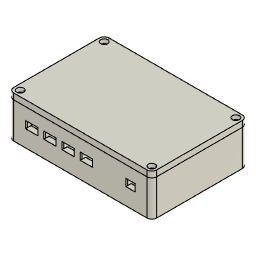
Box Innen v14 (Autodesk Fusion 360 design; units mm, degrees)
Autodesk Fusion 360 part; units mm, degrees
note: some values were not read from the file. Chosen so that the rebuilt part matches the saved one: which face or edge a step refers to.
sketch "Skizze5" plane through (0, 0, 0) normal (0, 0, 1) x (1, 0, 0)
  line L0 (60, -40) -> (-60, -40)
  line L1 (-60, -40) -> (-60, 40)
  line L2 (-60, 40) -> (60, 40)
  line L3 (60, 40) -> (60, -40)
  line L4 (60, -40) -> (-60, 40) construction
  line L5 (-60, -40) -> (60, 40) construction
  dimension "d11" = 120
  dimension "d12" = 80
  constraint perpendicular L0 L1
  constraint parallel L0 L2
  constraint parallel L1 L3
  constraint horizontal L0
  constraint coincident L4 origin
  constraint coincident L5 origin
  measures "d11" distance of L1.end L2.end
  measures "d12" distance of L0.end L1.end
extrude "Extrusion3" add sketch "Skizze5" along normal blind 30 makes body 1
sketch "Skizze6" plane through (0, 0, 30) normal (0, 0, 1) x (-1, 0, 0)
  line L0 (-60, -40) -> (60, -40)
  line L1 (60, -40) -> (60, 40)
  line L2 (60, 40) -> (-60, 40)
  line L3 (-60, 40) -> (-60, -40)
  line L4 (50.5, -38.5) -> (-50.5, -38.5)
  line L5 (-58.5, -30.5) -> (-58.5, 30.5)
  line L6 (-50.5, 38.5) -> (50.5, 38.5)
  line L7 (58.5, 30.5) -> (58.5, -30.5)
  line L8 (-50.5, -38.5) -> (-50.5, -30.5)
  line L9 (-50.5, -30.5) -> (-58.5, -30.5)
  line L10 (-58.5, 30.5) -> (-50.5, 30.5)
  line L11 (-50.5, 30.5) -> (-50.5, 38.5)
  line L12 (50.5, 38.5) -> (50.5, 30.5)
  line L13 (50.5, 30.5) -> (58.5, 30.5)
  line L14 (58.5, -30.5) -> (50.5, -30.5)
  line L15 (50.5, -30.5) -> (50.5, -38.5)
  line L16 (0, -75) -> (0, 75) construction
  line L17 (100, 0) -> (-100, 0) construction
  dimension "d15" = 1.5
  dimension "d16" = 1.5
  dimension "d26" = 8
  dimension "d27" = 8
  constraint perpendicular L1 L4
  constraint perpendicular L4 L5
  constraint perpendicular L5 L6
  constraint perpendicular L6 L7
  constraint perpendicular L4 L8
  constraint perpendicular L5 L9
  constraint perpendicular L5 L10
  constraint perpendicular L6 L12
  constraint perpendicular L7 L14
  constraint perpendicular L7 L13
  constraint perpendicular L6 L11
  constraint perpendicular L4 L15
  constraint perpendicular L6 L16
  constraint horizontal L17
  constraint symmetric L4.start L4.end L16
  constraint symmetric L5.start L7.end L16
  constraint symmetric L7.start L7.end L17
  constraint symmetric L4.start L6.end L17
  constraint symmetric L4.end L6.start L17
  constraint midpoint origin L17
  constraint midpoint origin L16
  constraint symmetric L5.start L5.end L17
  measures "d15" distance of L0 L4.end
  measures "d16" distance of L3 L5.start
  measures "d26" distance of L4.end L8.end
  measures "d27" distance of L5.start L8.end
extrude "Extrusion4" cut sketch "Skizze6" against normal blind 28 contours L4 L5 L6 L7 L8 L9 L10 L11 L12 L13 L14 L15 bodies 1
sketch "Skizze8" plane through (0, 0, 30) normal (0, 0, 1) x (-1, 0, 0)
  line L0 (58.5, 30.5) -> (58.5, -30.5)
  line L1 (58.5, -30.5) -> (50.5, -30.5)
  line L2 (50.5, -30.5) -> (50.5, -38.5)
  line L3 (50.5, -38.5) -> (-50.5, -38.5)
  line L4 (-50.5, -38.5) -> (-50.5, -30.5)
  line L5 (-50.5, -30.5) -> (-58.5, -30.5)
  line L6 (-58.5, -30.5) -> (-58.5, 30.5)
  line L7 (-58.5, 30.5) -> (-50.5, 30.5)
  line L8 (-50.5, 30.5) -> (-50.5, 38.5)
  line L9 (-50.5, 38.5) -> (50.5, 38.5)
  line L10 (50.5, 38.5) -> (50.5, 30.5)
  line L11 (50.5, 30.5) -> (58.5, 30.5)
  line L12 (-60, -40) -> (60, -40)
  line L13 (60, -40) -> (60, 40)
  line L14 (60, 40) -> (-60, 40)
  line L15 (-60, 40) -> (-60, -40)
  circle A0 centre (-55.25, -35.25) radius 1.7
  line L16 (-50.5, -30.5) -> (-60, -40) construction
  line L17 (80, 0) -> (-80, 0) construction
  line L18 (0, 55) -> (0, -55) construction
  circle A1 centre (55.25, -35.25) radius 1.7
  circle A2 centre (55.25, 35.25) radius 1.7
  circle A3 centre (-55.25, 35.25) radius 1.7
  line L19 (50.5, -30.5) -> (60, -40) construction
  line L20 (50.5, 30.5) -> (60, 40) construction
  line L21 (-50.5, 30.5) -> (-60, 40) construction
  point P0 (-55.25, -35.25)
  point P1 (55.25, -35.25)
  point P2 (55.25, 35.25)
  point P3 (-55.25, 35.25)
  dimension "d19" = 3.4
  dimension "d21" = 3.4
  dimension "d22" = 3.4
  dimension "d23" = 3.4
  constraint coincident L4.end L5.start
  constraint coincident L12.start L15.end
  constraint midpoint L16 P0
  constraint coincident P0 A0.centre
  constraint horizontal L17
  constraint perpendicular L3 L18
  constraint coincident L1.end L2.start
  constraint coincident L12.end L13.start
  constraint coincident L10.end L11.start
  constraint coincident L13.end L14.start
  constraint coincident L7.end L8.start
  constraint coincident L14.end L15.start
  constraint midpoint L19 P1
  constraint midpoint L20 P2
  constraint midpoint L21 P3
  constraint coincident P3 A3.centre
  constraint coincident P2 A2.centre
  constraint coincident P1 A1.centre
  measures "d19" diameter of A0
  measures "d21" diameter of A1
  measures "d22" diameter of A2
  measures "d23" diameter of A3
extrude "Extrusion6" cut sketch "Skizze8" against normal blind 30 contours A0 | A1 | A2 | A3 bodies 1
extrude "Extrusion7" cut sketch "Skizze8" against normal blind 28.5 contours L0 L1 L2 L3 L4 L5 L6 L7 L8 L9 L10 L11 bodies 1
sketch "Nuts" plane through (0, 0, 0) normal (0, 0, -1) x (1, 0, 0)
  line L0 (-60, -40) -> (60, -40)
  line L1 (60, -40) -> (60, 40)
  line L2 (60, 40) -> (-60, 40)
  line L3 (-60, 40) -> (-60, -40)
  line L4 (58.45, 33.4025) -> (58.45, 37.0975)
  line L5 (58.45, 37.0975) -> (55.25, 38.945)
  line L6 (55.25, 38.945) -> (52.05, 37.0975)
  line L7 (52.05, 37.0975) -> (52.05, 33.4025)
  line L8 (52.05, 33.4025) -> (55.25, 31.555)
  line L9 (55.25, 31.555) -> (58.45, 33.4025)
  line L10 (50.5, 30.5) -> (60, 40) construction
  line L11 (-55.25, 31.555) -> (-52.05, 33.4025)
  line L12 (-55.25, 38.945) -> (-58.45, 37.0975)
  line L13 (-58.45, 37.0975) -> (-58.45, 33.4025)
  line L14 (-52.05, 37.0975) -> (-55.25, 38.945)
  line L15 (-58.45, 33.4025) -> (-55.25, 31.555)
  line L16 (-52.05, 33.4025) -> (-52.05, 37.0975)
  line L17 (-58.45, -33.4025) -> (-58.45, -37.0975)
  line L18 (-55.25, -38.945) -> (-52.05, -37.0975)
  line L19 (-58.45, -37.0975) -> (-55.25, -38.945)
  line L20 (-52.05, -37.0975) -> (-52.05, -33.4025)
  line L21 (-55.25, -31.555) -> (-58.45, -33.4025)
  line L22 (-52.05, -33.4025) -> (-55.25, -31.555)
  line L23 (52.05, -37.0975) -> (55.25, -38.945)
  line L24 (58.45, -37.0975) -> (58.45, -33.4025)
  line L25 (58.45, -33.4025) -> (55.25, -31.555)
  line L26 (55.25, -31.555) -> (52.05, -33.4025)
  line L27 (52.05, -33.4025) -> (52.05, -37.0975)
  line L28 (55.25, -38.945) -> (58.45, -37.0975)
  line L29 (25, -40) -> (145, -40)
  line L30 (0, 55) -> (0, -55)
  line L31 (-100, 0) -> (100, 0)
  line L32 (0, -75) -> (0, 75)
  circle A0 centre (55.25, -35.25) radius 1.7
  circle A1 centre (55.25, 35.25) radius 1.7
  circle A2 centre (-55.25, -35.25) radius 1.7
  circle A3 centre (-55.25, 35.25) radius 1.7
  point P0 (55.25, 35.25)
  point P1 (55.25, 35.25)
  point P2 (50.5, 30.5)
  point P3 (55.25, 35.25)
  point P4 (-55.25, 35.25)
  point P5 (-55.25, 35.25)
  point P6 (-55.25, -35.25)
  point P7 (-55.25, -35.25)
  point P8 (55.25, -35.25)
  point P9 (55.25, -35.25)
  dimension "d35" = 3.2
  dimension "d36" = 3.2
  dimension "d37" = 3.2
  dimension "d38" = 3.2
  constraint coincident L1.end L2.start
  constraint midpoint L10 P3
  constraint coincident P3 P1
  constraint coincident P2 L10.start
  constraint coincident P5 P4
  constraint coincident P7 P6
  constraint coincident P9 P8
  constraint symmetric P3 P5 L30
  constraint symmetric P3 P9 L31
  constraint symmetric P5 P7 L31
  constraint parallel L27 L30
  constraint parallel L20 L32
  constraint parallel L16 L30
  constraint parallel L7 L32
  measures "d35" distance of P3 L4
  measures "d36" distance of P5 L16
  measures "d37" distance of P7 L20
  measures "d38" distance of P9 L24
extrude "Extrude8" cut sketch "Nuts" against normal blind 5 contours L4 L5 L6 L7 L8 L9 | L11 L12 L13 L14 L15 L16 | L17 L18 L19 L20 L21 L22 | L23 L24 L25 L26 L27 L28 | A0 | A1 | A2 | A3 bodies 1
sketch "Overhang long 1" plane through (0, -38.5, 0) normal (0, 1, 0) x (-1, 0, 0)
  line L0 (50.5, 30) -> (-50.5, 30)
  line L1 (-50.5, 30) -> (-50.5, 1.5)
  line L2 (-50.5, 1.5) -> (50.5, 1.5)
  line L3 (50.5, 1.5) -> (50.5, 30)
  line L4 (-50.5, 28) -> (50.5, 28)
  line L5 (50.5, 30) -> (-50.5, 30)
  dimension "d41" = 2
  constraint coincident L1 L4.start
  constraint coincident L3 L4.end
  constraint perpendicular L3 L4
  constraint coincident L0.start L3.end
  constraint coincident L0.end L1.start
  measures "d41" distance of L4.start L0.end
extrude "Extrude9" add sketch "Overhang long 1" along normal blind 3 contours L0 L1 L3 L4 L5 bodies 1
chamfer "Chamfer1" distance 2 angle 45 1 edges at (0, -35.5, 28) on bodies 1
sketch "Overhang short 1" plane through (-58.5, 0, 0) normal (1, 0, 0) x (0, 1, 0)
  line L0 (30.5, 30) -> (-30.5, 30)
  line L1 (-30.5, 30) -> (-30.5, 1.5)
  line L2 (-30.5, 1.5) -> (30.5, 1.5)
  line L3 (30.5, 1.5) -> (30.5, 30)
  line L4 (-30.5, 30) -> (30.5, 30)
  line L5 (30.5, 28) -> (-30.5, 28)
  dimension "d46" = 2
  constraint coincident L0.end L1.start
  constraint coincident L0.start L3.end
  constraint coincident L3 L5.start
  constraint coincident L1 L5.end
  constraint perpendicular L1 L5
  measures "d46" distance of L0.end L5.end
extrude "Extrude12" add sketch "Overhang short 1" along normal blind 3 contours L0 L1 L3 L4 L5 bodies 1
chamfer "Chamfer3" distance 2 angle 45 1 edges at (-55.5, 0, 28) on bodies 1
sketch "Overhang long 2" plane through (0, 38.5, 0) normal (0, -1, 0) x (1, 0, 0)
  line L0 (50.5, 30) -> (-50.5, 30)
  line L1 (-50.5, 30) -> (-50.5, 1.5)
  line L2 (-50.5, 1.5) -> (50.5, 1.5)
  line L3 (50.5, 1.5) -> (50.5, 30)
  line L4 (-50.5, 30) -> (50.5, 30)
  line L5 (50.5, 28) -> (-50.5, 28)
  dimension "d56" = 2
  constraint coincident L0.end L1.start
  constraint coincident L0.start L3.end
  constraint coincident L3 L5.start
  constraint coincident L1 L5.end
  constraint perpendicular L1 L5
  measures "d56" distance of L0.end L5.end
extrude "Extrude13" add sketch "Overhang long 2" along normal blind 3 contours L0 L1 L3 L4 L5 bodies 1
chamfer "Chamfer4" distance 2 angle 45 1 edges at (0, 35.5, 28) on bodies 1
sketch "Overhang short 2" plane through (58.5, 0, 0) normal (-1, 0, 0) x (0, -1, 0)
  line L0 (30.5, 30) -> (-30.5, 30)
  line L1 (-30.5, 30) -> (-30.5, 1.5)
  line L2 (-30.5, 1.5) -> (30.5, 1.5)
  line L3 (30.5, 1.5) -> (30.5, 30)
  line L4 (-30.5, 30) -> (30.5, 30)
  line L5 (30.5, 28) -> (-30.5, 28)
  dimension "d60" = 2
  constraint coincident L0.end L1.start
  constraint coincident L0.start L3.end
  constraint coincident L3 L5.start
  constraint coincident L1 L5.end
  constraint perpendicular L1 L5
  measures "d60" distance of L0.end L5.end
extrude "Extrude14" add sketch "Overhang short 2" along normal blind 3 contours L0 L1 L3 L4 L5 bodies 1
chamfer "Chamfer5" distance 2 angle 45 1 edges at (55.5, 0, 28) on bodies 1
sketch "Sealing" plane through (0, 0, 30) normal (0, 0, 1) x (-1, 0, 0)
  circle A0 centre (-55.25, -35.25) radius 1.7
  circle A1 centre (-55.25, 35.25) radius 1.7
  circle A2 centre (55.25, -35.25) radius 1.7
  circle A3 centre (55.25, 35.25) radius 1.7
  line L0 (55.5, -30.5) -> (50.5, -30.5)
  line L1 (50.5, -30.5) -> (50.5, -35.5)
  line L2 (50.5, -35.5) -> (-50.5, -35.5)
  line L3 (-50.5, -35.5) -> (-50.5, -30.5)
  line L4 (-50.5, -30.5) -> (-55.5, -30.5)
  line L5 (-55.5, -30.5) -> (-55.5, 30.5)
  line L6 (-55.5, 30.5) -> (-50.5, 30.5)
  line L7 (-50.5, 30.5) -> (-50.5, 35.5)
  line L8 (-50.5, 35.5) -> (50.5, 35.5)
  line L9 (50.5, 35.5) -> (50.5, 30.5)
  line L10 (50.5, 30.5) -> (55.5, 30.5)
  line L11 (55.5, 30.5) -> (55.5, -30.5)
  line L12 (-60, -40) -> (60, -40)
  line L13 (60, -40) -> (60, 40)
  line L14 (60, 40) -> (-60, 40)
  line L15 (-60, 40) -> (-60, -40)
  line L16 (50.5, -35.5) -> (-50.5, -35.5)
  line L17 (-50.5, -30.5) -> (-55.5, -30.5)
  line L18 (-55.5, 30.5) -> (-50.5, 30.5)
  line L19 (-50.5, 35.5) -> (50.5, 35.5)
  line L20 (50.5, 30.5) -> (55.5, 30.5)
  line L21 (55.5, -30.5) -> (50.5, -30.5)
  line L22 (50.5, -36.5) -> (-50.5, -36.5)
  line L23 (-50.5, -36.5) -> (-51.5, -35.5)
  line L24 (-51.5, -35.5) -> (-51.5, -31.5)
  line L25 (-51.5, -31.5) -> (-55.5, -31.5)
  line L26 (-55.5, -31.5) -> (-56.5, -30.5)
  line L27 (-56.5, -30.5) -> (-56.5, 30.5)
  line L28 (-56.5, 30.5) -> (-55.5, 31.5)
  line L29 (-55.5, 31.5) -> (-51.5, 31.5)
  line L30 (-51.5, 31.5) -> (-51.5, 35.5)
  line L31 (-51.5, 35.5) -> (-50.5, 36.5)
  line L32 (-50.5, 36.5) -> (50.5, 36.5)
  line L33 (50.5, 36.5) -> (51.5, 35.5)
  line L34 (51.5, 35.5) -> (51.5, 31.5)
  line L35 (51.5, 31.5) -> (55.5, 31.5)
  line L36 (55.5, 31.5) -> (56.5, 30.5)
  line L37 (56.5, 30.5) -> (56.5, -30.5)
  line L38 (56.5, -30.5) -> (55.5, -31.5)
  line L39 (55.5, -31.5) -> (51.5, -31.5)
  line L40 (51.5, -31.5) -> (51.5, -35.5)
  line L41 (51.5, -35.5) -> (50.5, -36.5)
  line L42 (0, -75) -> (0, 75) construction
  line L43 (100, 0) -> (-100, 0) construction
  dimension "d64" = 1
  dimension "d65" = 1
  dimension "d66" = 1
  dimension "d67" = 1
  dimension "d68" = 1
  dimension "d69" = 1
  constraint coincident L1.end L2.start
  constraint coincident L2.end L3.start
  constraint coincident L3.end L4.start
  constraint coincident L4.end L5.start
  constraint coincident L5.end L6.start
  constraint coincident L6.end L7.start
  constraint coincident L7.end L8.start
  constraint coincident L8.end L9.start
  constraint coincident L9.end L10.start
  constraint coincident L10.end L11.start
  constraint coincident L0.start L11.end
  constraint coincident L0.end L1.start
  constraint perpendicular L3 L22
  constraint perpendicular L22 L24
  constraint perpendicular L24 L25
  constraint parallel L23 L26
  constraint perpendicular L25 L27
  constraint perpendicular L27 L29
  constraint perpendicular L29 L30
  constraint parallel L28 L31
  constraint parallel L14 L32
  constraint perpendicular L14 L34
  constraint perpendicular L34 L35
  constraint parallel L33 L36
  constraint parallel L13 L37
  constraint perpendicular L36 L38
  constraint perpendicular L37 L39
  constraint perpendicular L39 L40
  constraint coincident L16 L23.end
  constraint coincident L5 L25.end
  constraint coincident L17 L26.end
  constraint vertical L42
  constraint perpendicular L37 L43
  constraint symmetric L22.start L22.end L42
  constraint symmetric L23.end L40.end L42
  constraint symmetric L25.end L38.end L42
  constraint symmetric L26.end L37.end L42
  constraint symmetric L25.end L28.end L43
  constraint symmetric L26.end L27.end L43
  constraint symmetric L23.end L30.end L43
  constraint symmetric L22.end L31.end L43
  constraint symmetric L22.start L32.end L43
  constraint symmetric L33.end L40.end L43
  constraint symmetric L35.end L38.end L43
  constraint symmetric L36.end L37.end L43
  measures "d64" distance of L2.end L22.end
  measures "d65" distance of L2.end L23.end
  measures "d66" distance of L4.end L25.end
  measures "d67" distance of L4.end L26.end
  measures "d68" distance of L1.end L40.end
  measures "d69" distance of L10.end L35.end
extrude "Extrude15" add sketch "Sealing" along normal blind 2.7 contours L22 L23 L24 L25 L26 L27 L28 L29 L30 L31 L32 L33 L34 L35 L36 L37 L38 L39 L40 L41 bodies 1
sketch "Groove" plane through (0, 0, 30) normal (0, 0, 1) x (-1, 0, 0)
  line L0 (51.5, -35.5) -> (50.5, -36.5)
  line L1 (50.5, -36.5) -> (-50.5, -36.5)
  line L2 (-50.5, -36.5) -> (-51.5, -35.5)
  line L3 (-51.5, -35.5) -> (-51.5, -31.5)
  line L4 (-51.5, -31.5) -> (-55.5, -31.5)
  line L5 (-55.5, -31.5) -> (-56.5, -30.5)
  line L6 (-56.5, -30.5) -> (-56.5, 30.5)
  line L7 (-56.5, 30.5) -> (-55.5, 31.5)
  line L8 (-55.5, 31.5) -> (-51.5, 31.5)
  line L9 (-51.5, 31.5) -> (-51.5, 35.5)
  line L10 (-51.5, 35.5) -> (-50.5, 36.5)
  line L11 (-50.5, 36.5) -> (50.5, 36.5)
  line L12 (50.5, 36.5) -> (51.5, 35.5)
  line L13 (51.5, 35.5) -> (51.5, 31.5)
  line L14 (51.5, 31.5) -> (55.5, 31.5)
  line L15 (55.5, 31.5) -> (56.5, 30.5)
  line L16 (56.5, 30.5) -> (56.5, -30.5)
  line L17 (56.5, -30.5) -> (55.5, -31.5)
  line L18 (55.5, -31.5) -> (51.5, -31.5)
  line L19 (51.5, -31.5) -> (51.5, -35.5)
  circle A0 centre (-55.25, -35.25) radius 1.7
  circle A1 centre (-55.25, 35.25) radius 1.7
  circle A2 centre (55.25, -35.25) radius 1.7
  circle A3 centre (55.25, 35.25) radius 1.7
  line L20 (-60, -40) -> (60, -40)
  line L21 (60, -40) -> (60, 40)
  line L22 (60, 40) -> (-60, 40)
  line L23 (-60, 40) -> (-60, -40)
  line L24 (50.5, -36.5) -> (-50.5, -36.5)
  line L25 (-51.5, -35.5) -> (-51.5, -31.5)
  line L26 (-55.5, -31.5) -> (-56.5, -30.5)
  line L27 (-56.5, 30.5) -> (-55.5, 31.5)
  line L28 (-51.5, 31.5) -> (-51.5, 35.5)
  line L29 (-50.5, 36.5) -> (50.5, 36.5)
  line L30 (51.5, 35.5) -> (51.5, 31.5)
  line L31 (55.5, 31.5) -> (56.5, 30.5)
  line L32 (56.5, -30.5) -> (55.5, -31.5)
  line L33 (51.5, -31.5) -> (51.5, -35.5)
  line L34 (50.9971, -37.7) -> (-50.9971, -37.7)
  line L35 (-50.9971, -37.7) -> (-52.7, -35.9971)
  line L36 (-52.7, -35.9971) -> (-52.7, -32.7)
  line L37 (-52.7, -32.7) -> (-55.9971, -32.7)
  line L38 (-55.9971, -32.7) -> (-57.7, -30.9971)
  line L39 (-57.7, -30.9971) -> (-57.7, 30.9971)
  line L40 (-57.7, 30.9971) -> (-55.9971, 32.7)
  line L41 (-55.9971, 32.7) -> (-52.7, 32.7)
  line L42 (-52.7, 32.7) -> (-52.7, 35.9971)
  line L43 (-52.7, 35.9971) -> (-50.9971, 37.7)
  line L44 (-50.9971, 37.7) -> (50.9971, 37.7)
  line L45 (50.9971, 37.7) -> (52.7, 35.9971)
  line L46 (52.7, 35.9971) -> (52.7, 32.7)
  line L47 (52.7, 32.7) -> (55.9971, 32.7)
  line L48 (55.9971, 32.7) -> (57.7, 30.9971)
  line L49 (57.7, 30.9971) -> (57.7, -30.9971)
  line L50 (57.7, -30.9971) -> (55.9971, -32.7)
  line L51 (55.9971, -32.7) -> (52.7, -32.7)
  line L52 (52.7, -32.7) -> (52.7, -35.9971)
  line L53 (52.7, -35.9971) -> (50.9971, -37.7)
  line L54 (-50.5, -30.5) -> (-52.7, -32.7) construction
  line L55 (0, -75) -> (0, 75) construction
  line L56 (100, 0) -> (-100, 0) construction
  line L57 (-100, 0) -> (-101.3533, 0) construction
  point P0 (-50.5, -30.5)
  dimension "d77" = 1.2
  dimension "d78" = 1.2
  dimension "d79" = 1.2
  dimension "d80" = 1.2
  dimension "d81" = 1.2
  dimension "d82" = 1.2
  constraint coincident L0.end L1.start
  constraint coincident L1.end L2.start
  constraint coincident L2.end L3.start
  constraint coincident L3.end L4.start
  constraint coincident L4.end L5.start
  constraint coincident L5.end L6.start
  constraint coincident L6.end L7.start
  constraint coincident L7.end L8.start
  constraint coincident L8.end L9.start
  constraint coincident L9.end L10.start
  constraint coincident L10.end L11.start
  constraint coincident L11.end L12.start
  constraint coincident L12.end L13.start
  constraint coincident L13.end L14.start
  constraint coincident L14.end L15.start
  constraint coincident L15.end L16.start
  constraint coincident L16.end L17.start
  constraint coincident L17.end L18.start
  constraint coincident L18.end L19.start
  constraint coincident L0.start L19.end
  constraint parallel L20 L34
  constraint perpendicular L36 L37
  constraint parallel L23 L39
  constraint perpendicular L23 L41
  constraint perpendicular L41 L42
  constraint parallel L40 L43
  constraint perpendicular L42 L44
  constraint perpendicular L43 L45
  constraint perpendicular L44 L46
  constraint perpendicular L46 L47
  constraint parallel L45 L48
  constraint parallel L21 L49
  constraint perpendicular L48 L50
  constraint perpendicular L21 L51
  constraint perpendicular L51 L52
  constraint collinear L3.end L36.end P0
  constraint equal L36 L37
  constraint coincident P0 L54.start
  constraint symmetric L34.end L38.end L54
  constraint vertical L55
  constraint horizontal L56
  constraint symmetric L34.start L34.end L55
  constraint symmetric L35.end L52.end L55
  constraint symmetric L37.end L50.end L55
  constraint symmetric L38.end L49.end L55
  constraint symmetric L38.end L39.end L56
  constraint symmetric L37.end L40.end L56
  constraint symmetric L35.end L42.end L56
  constraint symmetric L34.end L43.end L56
  constraint symmetric L39.end L48.end L55
  constraint symmetric L40.end L47.end L55
  constraint symmetric L42.end L45.end L55
  measures "d77" distance of L4 L37
  measures "d78" distance of L26 L38
  measures "d79" distance of L6 L39
  measures "d80" distance of L24 L34
  measures "d81" distance of L32 L50
  measures "d82" distance of L15.end L48
extrude "Extrude16" cut sketch "Groove" against normal blind 0.9 contours L34 L35 L36 L37 L38 L39 L40 L41 L42 L43 L44 L45 L46 L47 L48 L49 L50 L51 L52 L53 bodies 1
sketch "Lid Ground" plane through (0, 0, 30) normal (0, 0, 1) x (-1, 0, 0)
  line L0 (55.9971, -32.7) -> (52.7, -32.7)
  line L1 (52.7, -32.7) -> (52.7, -35.9971)
  line L2 (52.7, -35.9971) -> (50.9971, -37.7)
  line L3 (50.9971, -37.7) -> (-50.9971, -37.7)
  line L4 (-50.9971, -37.7) -> (-52.7, -35.9971)
  line L5 (-52.7, -35.9971) -> (-52.7, -32.7)
  line L6 (-52.7, -32.7) -> (-55.9971, -32.7)
  line L7 (-55.9971, -32.7) -> (-57.7, -30.9971)
  line L8 (-57.7, -30.9971) -> (-57.7, 30.9971)
  line L9 (-57.7, 30.9971) -> (-55.9971, 32.7)
  line L10 (-55.9971, 32.7) -> (-52.7, 32.7)
  line L11 (-52.7, 32.7) -> (-52.7, 35.9971)
  line L12 (-52.7, 35.9971) -> (-50.9971, 37.7)
  line L13 (-50.9971, 37.7) -> (50.9971, 37.7)
  line L14 (50.9971, 37.7) -> (52.7, 35.9971)
  line L15 (52.7, 35.9971) -> (52.7, 32.7)
  line L16 (52.7, 32.7) -> (55.9971, 32.7)
  line L17 (55.9971, 32.7) -> (57.7, 30.9971)
  line L18 (57.7, 30.9971) -> (57.7, -30.9971)
  line L19 (57.7, -30.9971) -> (55.9971, -32.7)
  circle A0 centre (-55.25, -35.25) radius 1.7
  circle A1 centre (-55.25, 35.25) radius 1.7
  circle A2 centre (55.25, -35.25) radius 1.7
  circle A3 centre (55.25, 35.25) radius 1.7
  line L20 (-60, -40) -> (60, -40)
  line L21 (60, -40) -> (60, 40)
  line L22 (60, 40) -> (-60, 40)
  line L23 (-60, 40) -> (-60, -40)
  line L24 (60, -40) -> (-60, -40)
  line L25 (-60, -40) -> (-60, 40)
  line L26 (-60, 40) -> (60, 40)
  line L27 (60, 40) -> (60, -40)
  constraint horizontal L24
  constraint vertical L25
  constraint horizontal L26
  constraint vertical L27
  constraint coincident L22.end L23.start
  constraint coincident L20.end L21.start
extrude "Extrude17" add sketch "Lid Ground" along normal blind 5 separate body makes body 2
delete_face "DeleteFace1" 20 faces at (-57.1324, 31.5647, 31.6667) (-57.7, -10.3324, 33.3333) (-56.5647, -32.1324, 31.6667) (-53.799, -32.7, 31.6667) (-52.7, -34.898, 31.6667) (-51.5647, -37.1324, 31.6667) (16.999, -37.7, 31.6667) (52.1324, -36.5647, 31.6667) (52.7, -33.799, 31.6667) (54.898, -32.7, 31.6667) (57.1324, -31.5647, 31.6667) (57.7, 10.3324, 33.3333) (56.5647, 32.1324, 31.6667) (53.799, 32.7, 31.6667) (52.7, 34.898, 31.6667) (51.5647, 37.1324, 31.6667) (-16.999, 37.7, 31.6667) (-52.1324, 36.5647, 31.6667) (-52.7, 33.799, 31.6667) (-54.898, 32.7, 31.6667) on bodies 2
sketch "Screw heads" plane through (0, 0, 35) normal (0, 0, 1) x (-1, 0, 0)
  circle A0 centre (55.25, -35.25) radius 1.7
  circle A1 centre (-55.25, 35.25) radius 1.7
  circle A2 centre (-55.25, -35.25) radius 1.7
  circle A3 centre (55.25, 35.25) radius 1.7
  line L0 (60, 40) -> (-60, 40)
  line L1 (-60, 40) -> (-60, -40)
  line L2 (-60, -40) -> (60, -40)
  line L3 (60, -40) -> (60, 40)
  circle A4 centre (55.25, -35.25) radius 2.95
  circle A5 centre (-55.25, -35.25) radius 2.95
  circle A6 centre (-55.25, 35.25) radius 2.95
  circle A7 centre (55.25, 35.25) radius 2.95
  dimension "d87" = 5.9
  dimension "d88" = 5.9
  dimension "d89" = 5.9
  dimension "d90" = 5.9
  constraint concentric A0 A4
  constraint concentric A2 A5
  constraint concentric A1 A6
  constraint concentric A3 A7
  measures "d87" diameter of A4
  measures "d88" diameter of A5
  measures "d89" diameter of A6
  measures "d90" diameter of A7
extrude "Extrude18" cut sketch "Screw heads" against normal blind 3.4 contours A4 | A5 | A6 | A7 bodies 2
sketch "Sealing groove" plane through (0, 0, 30) normal (0, 0, -1) x (1, 0, 0)
  line L0 (-60, -40) -> (60, -40)
  line L1 (60, -40) -> (60, 40)
  line L2 (60, 40) -> (-60, 40)
  line L3 (-60, 40) -> (-60, -40)
  line L4 (-50.6243, 36.8) -> (50.6243, 36.8)
  line L5 (50.6243, 36.8) -> (51.8, 35.6243)
  line L6 (51.8, 31.8) -> (55.6243, 31.8)
  line L7 (51.8, 35.6243) -> (51.8, 31.8)
  line L8 (55.6243, 31.8) -> (56.8, 30.6243)
  line L9 (56.8, 30.6243) -> (56.8, -30.6243)
  line L10 (56.8, -30.6243) -> (55.6243, -31.8)
  line L11 (55.6243, -31.8) -> (51.8, -31.8)
  line L12 (51.8, -31.8) -> (51.8, -35.6243)
  line L13 (50.6243, -36.8) -> (-50.6243, -36.8)
  line L14 (-50.6243, -36.8) -> (-51.8, -35.6243)
  line L15 (-51.8, -35.6243) -> (-51.8, -31.8)
  line L16 (-51.8, -31.8) -> (-55.6243, -31.8)
  line L17 (-56.8, -30.6243) -> (-56.8, 30.6243)
  line L18 (-56.8, 30.6243) -> (-55.6243, 31.8)
  line L19 (-51.8, 31.8) -> (-51.8, 35.6243)
  line L20 (-51.8, 35.6243) -> (-50.6243, 36.8)
  line L21 (-55.6243, 31.8) -> (-51.8, 31.8)
  line L22 (-55.6243, -31.8) -> (-56.8, -30.6243)
  line L23 (50.6243, -36.8) -> (51.8, -35.6243)
  line L24 (-100, 0) -> (100, 0) construction
  line L25 (0, -75) -> (0, 75) construction
  line L26 (-50.2, 35.2) -> (50.2, 35.2)
  line L27 (50.2, 35.2) -> (50.2, 30.2)
  line L28 (50.2, 30.2) -> (55.2, 30.2)
  line L29 (55.2, 30.2) -> (55.2, -30.2)
  line L30 (55.2, -30.2) -> (50.2, -30.2)
  line L31 (50.2, -30.2) -> (50.2, -35.2)
  line L32 (50.2, -35.2) -> (-50.2, -35.2)
  line L33 (-50.2, -35.2) -> (-50.2, -30.2)
  line L34 (-50.2, -30.2) -> (-55.2, -30.2)
  line L35 (-55.2, -30.2) -> (-55.2, 30.2)
  line L36 (-55.2, 30.2) -> (-50.2, 30.2)
  line L37 (-50.2, 30.2) -> (-50.2, 35.2)
  line L38 (-55.5, 30.5) -> (-55.5, -30.5) construction
  circle A0 centre (-55.25, -35.25) radius 1.7
  circle A1 centre (55.25, 35.25) radius 1.7
  circle A2 centre (55.25, -35.25) radius 1.7
  circle A3 centre (-55.25, 35.25) radius 1.7
  line L39 (60, 40) -> (-60, 40)
  line L40 (-60, 40) -> (-60, -40)
  line L41 (-60, -40) -> (60, -40)
  line L42 (60, -40) -> (60, 40)
  line L43 (51.5, 35.5) -> (50.5, 36.5)
  line L44 (55.5, 31.5) -> (51.5, 31.5)
  line L45 (51.5, 31.5) -> (51.5, 35.5)
  line L46 (56.5, -30.5) -> (56.5, 30.5)
  line L47 (50.5, 36.5) -> (-50.5, 36.5)
  line L48 (56.5, 30.5) -> (55.5, 31.5)
  line L49 (50.5, 35.5) -> (-50.5, 35.5)
  line L50 (55.5, 30.5) -> (50.5, 30.5)
  line L51 (50.5, 30.5) -> (50.5, 35.5) construction
  line L52 (55.5, 30.5) -> (55.5, -30.5) construction
  point P0 (55.5, 31.5)
  dimension "d101" = 0.3
  dimension "d102" = 1.6
  dimension "d104" = 0.3
  dimension "d105" = 0.3
  dimension "d106" = 0.3
  dimension "d107" = 0.3
  dimension "d108" = 0.3
  dimension "d109" = 0.3
  dimension "d110" = 0.3
  dimension "d111" = 0.3
  dimension "d112" = 0.3
  dimension "d113" = 0.3
  constraint perpendicular L6 L7
  constraint parallel L1 L9
  constraint horizontal L11
  constraint perpendicular L11 L12
  constraint perpendicular L15 L16
  constraint perpendicular L16 L17
  constraint parallel L17 L19
  constraint perpendicular L19 L21
  constraint coincident L6.start L7.end
  constraint symmetric L8.end L9.end L24
  constraint symmetric L6.end L10.end L24
  constraint symmetric L5.end L12.end L24
  constraint symmetric L4.end L13.start L24
  constraint symmetric L4.start L4.end L25
  constraint symmetric L5.end L19.end L25
  constraint symmetric L8.end L17.end L25
  constraint symmetric L6.end L25 L18.end
  constraint coincident L18.end L21.start
  constraint symmetric L9.end L17.start L25
  constraint coincident L17.start L22.end
  constraint symmetric L10.end L16.end L25
  constraint symmetric L13.start L13.end L25
  constraint symmetric L12.end L14.end L25
  constraint perpendicular L26 L27
  constraint perpendicular L27 L28
  constraint perpendicular L28 L29
  constraint perpendicular L29 L30
  constraint perpendicular L30 L31
  constraint perpendicular L31 L32
  constraint perpendicular L32 L33
  constraint perpendicular L33 L34
  constraint perpendicular L34 L35
  constraint perpendicular L33 L36
  constraint perpendicular L26 L37
  constraint symmetric L25 L27 L37
  constraint symmetric L24 L34 L36
  constraint symmetric L24 L26 L32
  constraint symmetric L24 L33 L37
  constraint symmetric L25 L28 L36
  constraint symmetric L25 L30 L34
  constraint parallel L8 L48
  constraint coincident L50.end L51.start
  constraint coincident L49.start L51.end
  constraint coincident L50.start L52.start
  constraint perpendicular L30 L52
  measures "d101" distance of L35 L38
  measures "d102" distance of L17 L35
  measures "d104" distance of L8 P0
  measures "d105" distance of L5 L43
  measures "d106" distance of L6 L44
  measures "d107" distance of L7 L45
  measures "d108" distance of L9 L46
  measures "d109" distance of L4 L47
  measures "d110" distance of L26 L49
  measures "d111" distance of L28 L50
  measures "d112" distance of L27 L51
  measures "d113" distance of L29 L52
extrude "Extrude20" cut sketch "Sealing groove" against normal blind 3 contours L4 L5 L6 L7 L8 L9 L10 L11 L12 L13 L14 L15 L16 L17 L18 L19 L20 L21 L22 L23 bodies 2
sketch "Lid inner" plane through (0, 0, 30) normal (0, 0, -1) x (1, 0, 0)
  line L0 (-50.2, 35.2) -> (-50.2, 30.2)
  line L1 (-50.2, 30.2) -> (-55.2, 30.2)
  line L2 (-55.2, 30.2) -> (-55.2, -30.2)
  line L3 (-55.2, -30.2) -> (-50.2, -30.2)
  line L4 (-50.2, -30.2) -> (-50.2, -35.2)
  line L5 (-50.2, -35.2) -> (50.2, -35.2)
  line L6 (50.2, -35.2) -> (50.2, -30.2)
  line L7 (50.2, -30.2) -> (55.2, -30.2)
  line L8 (55.2, -30.2) -> (55.2, 30.2)
  line L9 (55.2, 30.2) -> (50.2, 30.2)
  line L10 (50.2, 30.2) -> (50.2, 35.2)
  line L11 (50.2, 35.2) -> (-50.2, 35.2)
  line L12 (-49.2, 34.2) -> (49.2, 34.2)
  line L13 (49.2, 34.2) -> (49.2, 29.2)
  line L14 (49.2, 29.2) -> (54.2, 29.2)
  line L15 (54.2, 29.2) -> (54.2, -29.2)
  line L16 (54.2, -29.2) -> (49.2, -29.2)
  line L17 (49.2, -29.2) -> (49.2, -34.2)
  line L18 (49.2, -34.2) -> (-49.2, -34.2)
  line L19 (-49.2, -34.2) -> (-49.2, -29.2)
  line L20 (-49.2, -29.2) -> (-54.2, -29.2)
  line L21 (-54.2, -29.2) -> (-54.2, 29.2)
  line L22 (-54.2, 29.2) -> (-49.2, 29.2)
  line L23 (-49.2, 29.2) -> (-49.2, 34.2)
  line L24 (0, -75) -> (0, 75) construction
  line L25 (-100, 0) -> (100, 0) construction
  dimension "d118" = 1
  dimension "d119" = 1
  dimension "d120" = 1
  dimension "d121" = 1
  constraint perpendicular L0 L12
  constraint perpendicular L12 L13
  constraint perpendicular L13 L14
  constraint perpendicular L7 L15
  constraint perpendicular L15 L16
  constraint perpendicular L7 L17
  constraint perpendicular L17 L18
  constraint perpendicular L18 L19
  constraint perpendicular L19 L20
  constraint perpendicular L18 L21
  constraint perpendicular L21 L22
  constraint perpendicular L12 L23
  constraint symmetric L14 L22 L24
  constraint symmetric L20 L22 L25
  constraint symmetric L12 L18 L25
  constraint symmetric L14 L16 L25
  constraint symmetric L13 L17 L25
  constraint symmetric L19 L23 L25
  measures "d118" distance of L11 L12
  measures "d119" distance of L10 L13
  measures "d120" distance of L9 L14
  measures "d121" distance of L8 L15
extrude "Extrude21" cut sketch "Lid inner" against normal blind 3 contours L12 L13 L14 L15 L16 L17 L18 L19 L20 L21 L22 L23 bodies 2
fillet "Fillet1" radius 4 1 edges at (-60, -40, 15) on bodies 1
fillet "Fillet2" radius 4 1 edges at (-60, 40, 15) on bodies 1
fillet "Fillet3" radius 4 1 edges at (60, 40, 15) on bodies 1
fillet "Fillet4" radius 4 1 edges at (60, -40, 15) on bodies 1
fillet "Fillet5" radius 4 1 edges at (60, -40, 32.5) on bodies 2
fillet "Fillet6" radius 4 1 edges at (-60, -40, 32.5) on bodies 2
fillet "Fillet7" radius 4 1 edges at (-60, 40, 32.5) on bodies 2
fillet "Fillet8" radius 4 1 edges at (60, 40, 32.5) on bodies 2
sketch "JST XH connectors" plane through (0, -40, 0) normal (0, -1, 0) x (1, 0, 0)
  line L0 (56, 0) -> (56, 30)
  line L1 (56, 30) -> (-56, 30)
  line L2 (-56, 30) -> (-56, 0)
  line L3 (-56, 0) -> (56, 0)
  line L4 (-35.7, 13.9817) -> (-46, 13.9817)
  line L5 (-46, 13.9817) -> (-46, 19.9817)
  line L6 (-46, 19.9817) -> (-35.7, 19.9817)
  line L7 (-35.7, 19.9817) -> (-35.7, 13.9817)
  line L8 (-35.7, 13.9817) -> (-46, 19.9817) construction
  line L9 (-46, 13.9817) -> (-35.7, 19.9817) construction
  line L10 (-56, 16.9788) -> (56, 17) construction
  line L11 (-20.4, 13.9846) -> (-30.7, 13.9846)
  line L12 (-20.4, 19.9846) -> (-20.4, 13.9846)
  line L13 (-30.7, 19.9846) -> (-20.4, 19.9846)
  line L14 (-30.7, 13.9846) -> (-30.7, 19.9846)
  line L15 (-20.4, 13.9846) -> (-30.7, 19.9846) construction
  line L16 (-30.7, 13.9846) -> (-20.4, 19.9846) construction
  line L17 (-5.1, 13.9874) -> (-15.4, 13.9874)
  line L18 (-5.1, 19.9874) -> (-5.1, 13.9874)
  line L19 (-15.4, 19.9874) -> (-5.1, 19.9874)
  line L20 (-15.4, 13.9874) -> (-5.1, 19.9874) construction
  line L21 (-5.1, 13.9874) -> (-15.4, 19.9874) construction
  line L22 (-15.4, 13.9874) -> (-15.4, 19.9874)
  line L23 (10.2, 13.9903) -> (-0.1, 13.9903)
  line L24 (10.2, 19.9903) -> (10.2, 13.9903)
  line L25 (-0.1, 19.9903) -> (10.2, 19.9903)
  line L26 (-0.1, 13.9903) -> (10.2, 19.9903) construction
  line L27 (10.2, 13.9903) -> (-0.1, 19.9903) construction
  line L28 (-0.1, 13.9903) -> (-0.1, 19.9903)
  line L29 (46, 19.9974) -> (46, 13.9974)
  line L30 (38.2, 19.9974) -> (46, 19.9974)
  line L31 (38.2, 13.9974) -> (38.2, 19.9974)
  line L32 (46, 13.9974) -> (38.2, 13.9974)
  line L33 (46, 13.9974) -> (38.2, 19.9974) construction
  line L34 (38.2, 13.9974) -> (46, 19.9974) construction
  point P0 (-40.85, 16.9817)
  point P1 (-56, 16.9788)
  point P2 (56, 17)
  point P3 (-25.55, 16.9846)
  point P4 (-10.25, 16.9874)
  point P5 (5.05, 16.9903)
  point P6 (42.1, 16.9974)
  dimension "d134" = 6
  dimension "d135" = 10.3
  dimension "d136" = 10
  dimension "d138" = 6
  dimension "d139" = 10.3
  dimension "d140" = 5
  dimension "d141" = 6
  dimension "d142" = 10.3
  dimension "d143" = 6
  dimension "d144" = 10.3
  dimension "d145" = 5
  dimension "d146" = 5
  dimension "d147" = 6
  dimension "d148" = 7.8
  dimension "d149" = 10
  constraint perpendicular L4 L5
  constraint parallel L4 L6
  constraint parallel L5 L7
  constraint horizontal L4
  constraint coincident L8 P0
  constraint coincident L9 P0
  constraint midpoint L8 P0
  constraint coincident L2 P1
  constraint coincident L0 P2
  constraint coincident P1 L10.start
  constraint coincident P2 L10.end
  constraint coincident P0 L10
  constraint perpendicular L11 L14
  constraint parallel L11 L13
  constraint parallel L12 L14
  constraint horizontal L11
  constraint coincident P3 L15
  constraint coincident P3 L16
  constraint midpoint P3 L15
  constraint coincident L10 P3
  constraint perpendicular L17 L22
  constraint parallel L17 L19
  constraint parallel L18 L22
  constraint horizontal L17
  constraint coincident P4 L21
  constraint coincident P4 L20
  constraint midpoint P4 L21
  constraint perpendicular L23 L28
  constraint parallel L23 L25
  constraint parallel L24 L28
  constraint horizontal L23
  constraint coincident P5 L27
  constraint coincident P5 L26
  constraint midpoint P5 L27
  constraint coincident L10 P4
  constraint coincident L10 P5
  constraint perpendicular L31 L32
  constraint parallel L30 L32
  constraint parallel L29 L31
  constraint horizontal L32
  constraint coincident P6 L33
  constraint coincident P6 L34
  constraint midpoint P6 L33
  constraint coincident L10 P6
  measures "d134" distance of L4.end L5.end
  measures "d135" distance of L5.end L6.end
  measures "d136" distance of L2 L5
  measures "d138" distance of L13.start L11.end
  measures "d139" distance of L13.start L12.start
  measures "d140" distance of L7 L14
  measures "d141" distance of L19.start L17.end
  measures "d142" distance of L19.start L18.start
  measures "d143" distance of L25.start L23.end
  measures "d144" distance of L25.start L24.start
  measures "d145" distance of L12 L22
  measures "d146" distance of L18 L28
  measures "d147" distance of L31.start L30.start
  measures "d148" distance of L29.start L30.start
  measures "d149" distance of L0 L29
extrude "Extrude22" cut sketch "JST XH connectors" against normal blind 1.5 contours L4 L5 L6 L7 | L11 L12 L13 L14 | L17 L18 L19 L22 | L23 L24 L25 L28 | L29 L30 L31 L32 bodies 1
sketch "JST XH connector support" plane through (0, -38.5, 0) normal (0, 1, 0) x (-1, 0, 0)
  line L0 (5.1, 13.9874) -> (5.1, 19.9874)
  line L1 (5.1, 19.9874) -> (15.4, 19.9874)
  line L2 (15.4, 19.9874) -> (15.4, 13.9874)
  line L3 (15.4, 13.9874) -> (5.1, 13.9874)
  line L4 (20.4, 13.9846) -> (20.4, 19.9846)
  line L5 (20.4, 19.9846) -> (30.7, 19.9846)
  line L6 (30.7, 19.9846) -> (30.7, 13.9846)
  line L7 (30.7, 13.9846) -> (20.4, 13.9846)
  line L8 (-10.2, 13.9903) -> (-10.2, 19.9903)
  line L9 (-10.2, 19.9903) -> (0.1, 19.9903)
  line L10 (0.1, 19.9903) -> (0.1, 13.9903)
  line L11 (0.1, 13.9903) -> (-10.2, 13.9903)
  line L12 (46, 19.9817) -> (46, 13.9817)
  line L13 (46, 13.9817) -> (35.7, 13.9817)
  line L14 (35.7, 13.9817) -> (35.7, 19.9817)
  line L15 (35.7, 19.9817) -> (46, 19.9817)
  line L16 (-46, 19.9974) -> (-38.2, 19.9974)
  line L17 (-38.2, 19.9974) -> (-38.2, 13.9974)
  line L18 (-38.2, 13.9974) -> (-46, 13.9974)
  line L19 (-46, 13.9974) -> (-46, 19.9974)
  line L20 (50.5, 28) -> (-50.5, 28)
  line L21 (-50.5, 28) -> (-50.5, 1.5)
  line L22 (-50.5, 1.5) -> (50.5, 1.5)
  line L23 (50.5, 1.5) -> (50.5, 28)
  line L24 (-46, 13.9974) -> (-38.2, 13.9974)
  line L25 (-38.2, 13.9974) -> (-38.2, 10.9974)
  line L26 (-38.2, 10.9974) -> (-46, 10.9974)
  line L27 (-46, 10.9974) -> (-46, 13.9974)
  line L28 (-10.2, 13.9903) -> (0.1, 13.9903)
  line L29 (0.1, 13.9903) -> (0.1, 10.9903)
  line L30 (0.1, 10.9903) -> (-10.2, 10.9903)
  line L31 (-10.2, 10.9903) -> (-10.2, 13.9903)
  line L32 (5.1, 13.9874) -> (15.4, 13.9874)
  line L33 (15.4, 13.9874) -> (15.4, 10.9874)
  line L34 (15.4, 10.9874) -> (5.1, 10.9874)
  line L35 (5.1, 10.9874) -> (5.1, 13.9874)
  line L36 (20.4, 13.9846) -> (30.7, 13.9846)
  line L37 (30.7, 13.9846) -> (30.7, 10.9846)
  line L38 (30.7, 10.9846) -> (20.4, 10.9846)
  line L39 (20.4, 10.9846) -> (20.4, 13.9846)
  line L40 (35.7, 13.9817) -> (46, 13.9817)
  line L41 (46, 13.9817) -> (46, 10.9817)
  line L42 (46, 10.9817) -> (35.7, 10.9817)
  line L43 (35.7, 10.9817) -> (35.7, 13.9817)
  dimension "d152" = 3
  dimension "d153" = 3
  dimension "d154" = 3
  dimension "d155" = 3
  dimension "d156" = 3
  constraint horizontal L24
  constraint vertical L25
  constraint horizontal L26
  constraint vertical L27
  constraint coincident L18.end L19.start
  constraint horizontal L28
  constraint vertical L29
  constraint horizontal L30
  constraint vertical L31
  constraint coincident L8.start L11.end
  constraint horizontal L32
  constraint vertical L33
  constraint horizontal L34
  constraint vertical L35
  constraint coincident L0.start L3.end
  constraint horizontal L36
  constraint vertical L37
  constraint horizontal L38
  constraint vertical L39
  constraint coincident L4.start L7.end
  constraint horizontal L40
  constraint vertical L41
  constraint horizontal L42
  constraint vertical L43
  constraint coincident L13.end L14.start
  constraint collinear L2 L33
  constraint collinear L10 L29
  constraint collinear L17 L25
  constraint collinear L6 L37
  constraint collinear L12 L41
  measures "d152" distance of L17.end L25.end
  measures "d153" distance of L10.end L29.end
  measures "d154" distance of L2.end L33.end
  measures "d155" distance of L6.end L37.end
  measures "d156" distance of L12.end L41.end
extrude "Extrude23" add sketch "JST XH connector support" along normal blind 3 contours L3 L32 L33 L34 L35 | L7 L36 L37 L38 L39 | L11 L28 L29 L30 L31 | L13 L40 L41 L42 L43 | L18 L24 L25 L26 L27 bodies 1
chamfer "Chamfer6" distance 3 angle 45 5 edges at (42.1, -35.5, 10.9974) (5.05, -35.5, 10.9903) (-10.25, -35.5, 10.9874) (-25.55, -35.5, 10.9846) (-40.85, -35.5, 10.9817) on bodies 1
sketch "PCB M2x5 holders" plane through (0, 0, 1.5) normal (0, 0, 1) x (-1, 0, 0)
  line L0 (50.5, 30.5) -> (50.5, 38.5)
  line L1 (50.5, 38.5) -> (-50.5, 38.5)
  line L2 (-50.5, 38.5) -> (-50.5, 30.5)
  line L3 (-50.5, 30.5) -> (-58.5, 30.5)
  line L4 (-58.5, 30.5) -> (-58.5, -30.5)
  line L5 (-58.5, -30.5) -> (-50.5, -30.5)
  line L6 (-50.5, -30.5) -> (-50.5, -38.5)
  line L7 (-50.5, -38.5) -> (50.5, -38.5)
  line L8 (50.5, -38.5) -> (50.5, -30.5)
  line L9 (50.5, -30.5) -> (58.5, -30.5)
  line L10 (58.5, -30.5) -> (58.5, 30.5)
  line L11 (58.5, 30.5) -> (50.5, 30.5)
  circle A0 centre (50.5, -25.5) radius 2.5
  circle A1 centre (50.5, -25.5) radius 0.95
  circle A2 centre (50.5, -0.2) radius 0.95
  circle A3 centre (50.5, -0.2) radius 2.5
  circle A4 centre (-14.5, -25.5) radius 0.95
  circle A5 centre (-14.5, -25.5) radius 2.5
  circle A6 centre (-14.5, -0.2) radius 2.5
  circle A7 centre (-14.5, -0.2) radius 0.95
  line L12 (50.5, -25.5) -> (-14.5, -25.5) construction
  line L13 (-14.5, -25.5) -> (-14.5, -0.2) construction
  line L14 (-14.5, -0.2) -> (50.5, -0.2) construction
  line L15 (50.5, -0.2) -> (50.5, -25.5) construction
  line L16 (55.5, 30.5) -> (55.5, -30.5)
  line L17 (50.5, -35.5) -> (-50.5, -35.5)
  dimension "d160" = 5
  dimension "d161" = 1.9
  dimension "d162" = 5
  dimension "d163" = 1.9
  dimension "d164" = 5
  dimension "d165" = 1.9
  dimension "d166" = 5
  dimension "d167" = 1.9
  dimension "d170" = 65
  dimension "d171" = 25.3
  dimension "d172" = 5
  dimension "d173" = 10
  constraint concentric A0 A1
  constraint concentric A2 A3
  constraint concentric A4 A5
  constraint concentric A6 A7
  constraint horizontal L12
  constraint vertical L13
  constraint horizontal L14
  constraint vertical L15
  constraint coincident A0.centre A1.centre
  constraint coincident A4.centre A5.centre
  constraint coincident A2.centre A3.centre
  constraint coincident A6.centre A7.centre
  measures "d160" diameter of A0
  measures "d161" diameter of A1
  measures "d162" diameter of A3
  measures "d163" diameter of A2
  measures "d164" diameter of A5
  measures "d165" diameter of A4
  measures "d166" diameter of A6
  measures "d167" diameter of A7
  measures "d170" distance of A0.centre A4.centre
  measures "d171" distance of A0.centre A2.centre
  measures "d172" distance of L15 L16
  measures "d173" distance of L12 L17
extrude "Extrude24" add sketch "PCB M2x5 holders" along normal blind 5 contours A0 | A3 | A5 | A6 bodies 1
extrude "Extrude19" [rolled back] along distance -3 taper angle 0
extrude "Extrusion11" [suppressed]
extrude "Extrude10" [suppressed]
chamfer "Chamfer2" [suppressed]
sketch "Skizze12" plane through (0, 38.5, 0) normal (0, -1, 0) x (1, 0, 0)
  line L0 (50.5, 30) -> (-50.5, 30)
  line L1 (-50.5, 30) -> (-50.5, 1.5)
  line L2 (-50.5, 1.5) -> (50.5, 1.5)
  line L3 (50.5, 1.5) -> (50.5, 30)
  line L4 (-50.5, 30) -> (50.5, 30)
  line L5 (50.5, 28) -> (-50.5, 28)
  dimension "d50" = 2
  constraint coincident L0.end L1.start
  constraint coincident L0.start L3.end
  constraint coincident L3 L5.start
  constraint coincident L1 L5.end
  constraint perpendicular L1 L5
  measures "d50" distance of L0.end L5.end
extrude "Extrusion5" [suppressed]
extrude "Extrusion1" [suppressed]
extrude "Extrusion2" [suppressed]
sketch "Skizze3" plane through (0, 0, 33) normal (0, 0, 1) x (-1, 0, 0)
  line L0 (60, 0) -> (-60, 0)
  line L1 (-60, 0) -> (-60, -80)
  line L2 (-60, -80) -> (60, -80)
  line L3 (60, -80) -> (60, 0)
  line L4 (55.3098, -77.6107) -> (-55.3236, -77.6107)
  line L5 (-55.3236, -77.6107) -> (-58.9816, -70.169)
  line L6 (-58.9816, -70.169) -> (-58, -6)
  line L7 (-58, -6) -> (-54, -2)
  line L8 (-54, -2) -> (53.4847, -2)
  line L9 (53.4847, -2) -> (56.5997, -5.115)
  line L10 (56.5997, -5.115) -> (56.5997, -72.7965)
  line L11 (56.5997, -72.7965) -> (55.3098, -77.6107)
  dimension "d7" = 2
  dimension "d8" = 6
  dimension "d9" = 2
  dimension "d10" = 6
  constraint horizontal L4
  constraint perpendicular L1 L8
  constraint perpendicular L7 L9
  constraint perpendicular L8 L10
  measures "d7" distance of L0 L7.end
  measures "d8" distance of L1 L7.end
  measures "d9" distance of L1 L6.end
  measures "d10" distance of L0 L6.end
equation "d19 = d23"
equation "d21 = d19"
equation "d22 = d19"
equation "d27 = d26"
equation "d36 = d35"
equation "d37 = d35"
equation "d38 = d35"
equation "d64 = d65"
equation "d66 = d65"
equation "d67 = d65"
equation "d68 = d65"
equation "d69 = d65"
equation "d77 = d80"
equation "d78 = d80"
equation "d79 = d80"
equation "d81 = d80"
equation "d82 = d80"
equation "d89 = d88"
equation "d90 = d88"
equation "d101 = d104"
equation "d105 = d104"
equation "d106 = d104"
equation "d107 = d104"
equation "d108 = d104"
equation "d109 = d104"
equation "d110 = d104"
equation "d111 = d104"
equation "d112 = d104"
equation "d113 = d104"
equation "d119 = d118"
equation "d120 = d118"
equation "d121 = d118"
equation "d134 = 5.7 mm + 0.3 mm"
equation "d135 = 10 mm + 0.3 mm"
equation "d138 = 5.7 mm + 0.3 mm"
equation "d139 = 10 mm + 0.3 mm"
equation "d140 = d136 / 2"
equation "d141 = 5.7 mm + 0.3 mm"
equation "d142 = 10 mm + 0.3 mm"
equation "d143 = 5.7 mm + 0.3 mm"
equation "d144 = 10 mm + 0.3 mm"
equation "d145 = d140"
equation "d146 = d140"
equation "d147 = 5.7 mm + 0.3 mm"
equation "d148 = 7.5 mm + 0.3 mm"
equation "d149 = d136"
equation "d153 = d152"
equation "d154 = d152"
equation "d155 = d152"
equation "d156 = d152"
named bodies: "Box", "Lid"
